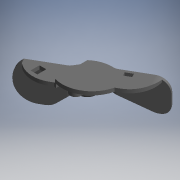
# Autodesk Inventor part: STOPPER-HSMCS50
Saved by Autodesk Inventor 2017.3 (Build 213256000, 256)
## iProperties
Part Number: STOPPER-HSMCS50
Material: Generic
Catalog Web Link: www.cadenas.de
Description: HSMC-STOPPER-Casters for Aluminum Frames-Corner Angle Type
Vendor: MISUMI
Document SubType Name: Modeling
Designer: partserver
Manufacturer: MISUMI
Mass: 4.89734 g
Surface Area: 50.4441 cm^2
Volume: 4.89734 cm^3
Density: 1 g/cm^3
Appearance: PSOLRGB-128-128-128
Category: PARTsolutions
Company: MISUMI
Title: STOPPER-HSMCS50
Author: Cadenas PARTsolutions
Comments: Casters for Aluminum Frames-Corner Angle Type
PSOL_IDENT_0: {$CADENAS_DATA\23d-libs\misumi\metric\39_accessories_for_al_extrusions\hsmcs_stopper.prj},176 {VTYP=
PSOL_IDENT_1: 3D},{NB=STOPPER-HSMCS50},{LINA=STOPPER-HSMCS50},{NN=HSMC-STOPPER},{DATE=30.06.2021 13:18:55},{GEOMDA
PSOL_IDENT_2: TE=25.03.2008 12:49:00},{VERSION=},{LINEID=60},{WBVAR=},{WBNUMERIC=}  {NB=STOPPER-HSMCS50},{LINA=STO
PSOL_IDENT_3: PPER-HSMCS50},{KT=DUMMY},{D=50},{TYPE=HSMCS},{AF=HFS5-2020},{H=70},{B=28},{DD=5.3},{E=27},{PN=STOPPE
PSOL_IDENT_4: R-HSMCS50},{RR=67},{HLP=1}
NB: STOPPER-HSMCS50
NN: HSMC-STOPPER
NT: Casters for Aluminum Frames-Corner Angle Type
NBSYN: $PN.
LINA: STOPPER-HSMCS50
CATALOG: Misumi
D: 50
TYPE: HSMCS
AF: HFS5-2020
H: 70
B: 28
DD: 5.3
E: 27
RR: 67
SUPPLIER: MISUMI
ARTICLENO: STOPPER-HSMCS50
BOMINFO: STOPPER-HSMCS50
CREATOR: CADENAS GmbH
Autodesk Inventor part; units mm, degrees
ref_plane "YZ Plane" through (0, 0, 0) normal (1, 0, 0) x (0, 1, 0)
ref_plane "XZ Plane" through (0, 0, 0) normal (0, 1, 0) x (-1, 0, 0)
ref_plane "XY Plane" through (0, 0, 0) normal (0, 0, 1) x (1, 0, 0)
sketch "Sketch_1" plane through (0, 0, 0) normal (0, 0, 1) x (1, 0, 0)
  line L0 (-28.4294, 25.5589) -> (-24.6062, 23.3516)
  arc A0 (-24.6062, 23.3516) -> (-16.9438, 4.0925) centre (-8.5838, 18.5724) ccw
  line L1 (-16.9438, 4.0925) -> (-14.9819, 2.9597)
  arc A1 (-14.5696, 2.4169) -> (-14.9819, 2.9597) centre (-15.4219, 2.1976) ccw
  arc A2 (-14.5696, 2.4169) -> (-13.7753, 0) centre (4.18, 7.24) ccw
  arc A3 (-13.7753, 0) -> (0, -11.6634) centre (4.18, 7.24) ccw
  arc A4 (0, -11.6634) -> (9.3779, -11.4092) centre (4.18, 7.24) ccw
  arc A5 (10.0541, -11.4948) -> (9.3779, -11.4092) centre (9.6141, -12.2569) ccw
  line L2 (10.0541, -11.4948) -> (12.0161, -12.6275)
  arc A6 (12.0161, -12.6275) -> (32.5262, -9.6338) centre (20.3761, 1.8524) ccw
  line L3 (32.5262, -9.6338) -> (36.3494, -11.8411)
  line L4 (36.3494, -11.8411) -> (37.2294, -10.3169)
  line L5 (37.2294, -10.3169) -> (15.1777, 2.4147)
  arc A7 (13.4621, 4.218) -> (15.1777, 2.4147) centre (17.3777, 6.2252) ccw
  arc A8 (13.4621, 4.218) -> (-3.0781, 13.7676) centre (-2.2, -3.8105) ccw
  arc A9 (-5.4977, 14.3516) -> (-3.0781, 13.7676) centre (-3.2977, 18.1621) ccw
  line L6 (-5.4977, 14.3516) -> (-27.5494, 27.0831)
  line L7 (-27.5494, 27.0831) -> (-28.4294, 25.5589)
  line L8 (19.8, -12.32) -> (24.2, -12.32)
  line L9 (24.2, -12.32) -> (24.2, -7.04)
  arc A10 (24.2, -7.04) -> (23.76, -6.6) centre (23.76, -7.04) ccw
  line L10 (23.76, -6.6) -> (20.24, -6.6)
  arc A11 (20.24, -6.6) -> (19.8, -7.04) centre (20.24, -7.04) ccw
  line L11 (19.8, -7.04) -> (19.8, -12.32)
  arc A12 (-14.2873, 14.8537) -> (-14.1263, 14.2526) centre (-13.9063, 14.6337) ccw
  line L12 (-14.1263, 14.2526) -> (-11.0778, 12.4926)
  arc A13 (-11.0778, 12.4926) -> (-10.4768, 12.6537) centre (-10.8578, 12.8737) ccw
  line L13 (-10.4768, 12.6537) -> (-9.3768, 14.5589)
  line L14 (-9.3768, 14.5589) -> (-13.1873, 16.7589)
  line L15 (-13.1873, 16.7589) -> (-14.2873, 14.8537)
  constraints: 32 end point, 28 point on circle, 14 centre point
extrude "Extrusion1" add sketch "Sketch_1" along normal blind 25
sketch "Sketch_2" plane through (0, 0, 2.3) normal (0, 0, 1) x (1, 0, 0)
  line L0 (-29.3094, 24.0347) -> (-25.4862, 21.8274)
  arc A0 (-25.4862, 21.8274) -> (-17.8238, 2.5683) centre (-9.4638, 17.0482) ccw
  line L1 (-17.8238, 2.5683) -> (-15.8619, 1.4355)
  arc A1 (-15.4496, 0.8927) -> (-15.8619, 1.4355) centre (-16.3019, 0.6734) ccw
  arc A2 (-15.4496, 0.8927) -> (-14.6553, -1.5242) centre (3.3, 5.7158) ccw
  arc A3 (-14.6553, -1.5242) -> (-0.88, -13.1876) centre (3.3, 5.7158) ccw
  arc A4 (-0.88, -13.1876) -> (8.4979, -12.9334) centre (3.3, 5.7158) ccw
  line L2 (8.4979, -12.9334) -> (8.4979, 7.921)
  arc A5 (8.4979, 7.921) -> (-3.9581, 12.2434) centre (-3.08, -5.3347) ccw
  arc A6 (-6.3777, 12.8274) -> (-3.9581, 12.2434) centre (-4.1777, 16.6379) ccw
  line L3 (-6.3777, 12.8274) -> (-28.4294, 25.5589)
  line L4 (-28.4294, 25.5589) -> (-29.3094, 24.0347)
  constraints: 14 point on circle, 10 end point, 7 centre point
extrude "Extrusion2" cut sketch "Sketch_2" along normal blind 50
sketch "Sketch_8" plane through (0, 0, 4.6) normal (0, 0, 1) x (1, 0, 0)
  line L0 (8.4979, 7.921) -> (8.4979, -12.9334)
  arc A0 (9.1741, -13.019) -> (8.4979, -12.9334) centre (8.7341, -13.7811) ccw
  line L1 (9.1741, -13.019) -> (11.1361, -14.1517)
  arc A1 (11.1361, -14.1517) -> (31.6462, -11.158) centre (19.4961, 0.3282) ccw
  line L2 (31.6462, -11.158) -> (35.4694, -13.3653)
  line L3 (35.4694, -13.3653) -> (36.3494, -11.8411)
  line L4 (36.3494, -11.8411) -> (14.2977, 0.8905)
  arc A2 (12.5821, 2.6938) -> (14.2977, 0.8905) centre (16.4977, 4.701) ccw
  arc A3 (12.5821, 2.6938) -> (8.4979, 7.921) centre (-3.08, -5.3347) ccw
  constraints: 10 end point, 8 point on circle, 4 centre point
extrude "Extrusion3" cut sketch "Sketch_8" along normal blind 50
sketch "Sketch_9" plane through (0, 0, 0) normal (0, 0, 1) x (1, 0, 0)
  line L0 (9.3779, 11.6892) -> (9.3779, -11.4092)
  arc A0 (10.0541, -11.4948) -> (9.3779, -11.4092) centre (9.6141, -12.2569) ccw
  line L1 (10.0541, -11.4948) -> (12.0161, -12.6275)
  arc A1 (12.0161, -12.6275) -> (32.5262, -9.6338) centre (20.3761, 1.8524) ccw
  line L2 (32.5262, -9.6338) -> (36.3494, -11.8411)
  line L3 (36.3494, -11.8411) -> (38.1094, -8.7927)
  line L4 (38.1094, -8.7927) -> (16.0577, 3.9389)
  arc A2 (14.3421, 5.7423) -> (16.0577, 3.9389) centre (18.2577, 7.7494) ccw
  arc A3 (14.3421, 5.7423) -> (9.3779, 11.6892) centre (-1.32, -2.2863) ccw
  line L5 (19.8, -12.32) -> (24.2, -12.32)
  line L6 (24.2, -12.32) -> (24.2, -7.04)
  arc A4 (24.2, -7.04) -> (23.76, -6.6) centre (23.76, -7.04) ccw
  line L7 (23.76, -6.6) -> (20.24, -6.6)
  arc A5 (20.24, -6.6) -> (19.8, -7.04) centre (20.24, -7.04) ccw
  line L8 (19.8, -7.04) -> (19.8, -12.32)
  constraints: 18 end point, 12 point on circle, 6 centre point
extrude "Extrusion4" cut sketch "Sketch_9" along normal blind 2.3
sketch "Sketch_3" plane through (0, 0, 0) normal (0.5, 0.8660254, 0) x (0.8660254, -0.5, 0)
  line L0 (-80, -90) -> (80, -90)
  line L1 (80, -90) -> (80, 10)
  line L2 (80, 10) -> (-80, 10)
  line L3 (-80, 10) -> (-80, -90)
  line L4 (-37.4, -8) -> (-37.4, -15)
  arc A0 (-37.4, -15) -> (-32.4, -20) centre (-32.4, -15) ccw
  line L5 (-32.4, -20) -> (-31.6329, -20)
  arc A1 (-31.6329, -20) -> (-28.8967, -19.5175) centre (-31.6329, -12) ccw
  line L6 (-28.8967, -19.5175) -> (-4.3403, -10.5797)
  arc A2 (3.5382, -11.9689) -> (-4.3403, -10.5797) centre (-1.6041, -18.0973) ccw
  line L7 (3.5382, -11.9689) -> (16.8375, -23.1284)
  arc A3 (16.8375, -23.1284) -> (21.9798, -25) centre (21.9798, -17) ccw
  line L8 (21.9798, -25) -> (25.4, -25)
  arc A4 (25.4, -25) -> (37.4, -13) centre (25.4, -13) ccw
  line L9 (37.4, -13) -> (37.4, -12)
  arc A5 (37.4, -12) -> (25.4, 0) centre (25.4, -12) ccw
  line L10 (25.4, 0) -> (-29.4, 0)
  arc A6 (-29.4, 0) -> (-37.4, -8) centre (-29.4, -8) ccw
  constraints: 22 end point, 14 point on circle, 7 centre point
extrude "Extrusion5" cut sketch "Sketch_3" along normal mid plane 100
sketch "Sketch_7" plane through (0, 0, 0) normal (1, 0, 0) x (0, 1, 0)
  line L0 (0, 0) -> (0, 8)
  line L1 (0, 8) -> (4, 8)
  arc A0 (6, 6) -> (4, 8) centre (4, 6) ccw
  line L2 (6, 6) -> (6, 5)
  line L3 (6, 5) -> (0, 5)
  line L4 (0, 5) -> (0, 8)
  constraints: 10 end point, 2 point on circle, 1 centre point
sketch "Sketch_4" plane through (0, 0, 2.3) normal (0, 0, 1) x (1, 0, 0)
  arc A0 (-3.5, -7.5) -> (3.5, -7.5) centre (0, -7.5) ccw
  line L0 (3.5, -7.5) -> (3.5, 7.5)
  arc A1 (3.5, 7.5) -> (-3.5, 7.5) centre (0, 7.5) ccw
  line L1 (-3.5, 7.5) -> (-3.5, -7.5)
  constraints: 4 end point, 4 point on circle, 2 centre point
extrude "Extrusion6" add sketch "Sketch_4" along normal blind 2.7
revolve "Revolution1" add sketch "Sketch_7" angle 360 about axis through (0, 0, 0) along (0, 0, -1)
ref_plane "stopper_to_body_XY" through (0, 0, 0) normal (0, 0, 1) x (1, 0, 0)
ref_plane "stopper_to_body_YZ" through (0, 0, 0) normal (1, 0, 0) x (0, 1, 0)
ref_plane "stopper_to_body_ZX" through (0, 0, 0) normal (0, 1, 0) x (0, 0, 1)
body "Solid1"
